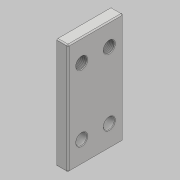
# Autodesk Inventor part: exercise3-3
Saved by Autodesk Inventor 2018 (Build 220112000, 112)
## iProperties
Created: 2020-09-23
Part Number: exercise3-3
Material: 一般
Document SubType Name: Modeling
Designer: 王鼎鈞
Density: 1 g/cm^3
Appearance: 預設
Author: 王鼎鈞
Autodesk Inventor part; units mm, degrees
ref_plane "YZ Plane" through (0, 0, 0) normal (1, 0, 0) x (0, 1, 0)
ref_plane "XZ Plane" through (0, 0, 0) normal (0, 1, 0) x (-1, 0, 0)
ref_plane "XY Plane" through (0, 0, 0) normal (0, 0, 1) x (1, 0, 0)
sketch "草圖1" plane through (0, 0, 0) normal (1, 0, 0) x (0, 1, 0)
  line L0 (-25, 50) -> (25, 50)
  line L1 (25, 50) -> (25, -50)
  line L2 (25, -50) -> (-25, -50)
  line L3 (-25, -50) -> (-25, 50)
  line L4 (-25, 50) -> (25, -50) construction
  line L5 (25, 50) -> (-25, -50) construction
  point P0 (0, 0)
  dimension "d0" = 50
  dimension "d1" = 100
  constraints: 12 end point, 2 midpoint, 2 parallel, 1 horizontal, 1 perpendicular
  measures "d0" distance of L1.end L2.end
  measures "d1" distance of L0.end L1.end
extrude "擠出1" add sketch "草圖1" along normal blind 10
fillet "圓角1" radius 1 4 edges at (5, 25, 50) (5, -25, 50) (5, 25, -50) (5, -25, -50)
chamfer "倒角1" distance 1 angle 45 8 edges at (10, -25, 0) (10, -24.7071, -49.7071) (10, 0, -50) (10, 24.7071, -49.7071) (10, 25, 0) (10, 24.7071, 49.7071) (10, 0, 50) (10, -24.7071, 49.7071)
sketch "草圖2" plane through (10, 0, 0) normal (1, 0, 0) x (0, 0, -1)
  line L0 (-50, 24) -> (-50, -24) projected
  line L1 (49, 25) -> (-49, 25) projected
  line L2 (-30, 24) -> (-30, -24)
  line L3 (50, -24) -> (50, 24) projected
  line L4 (30, -24) -> (30, 24)
  line L5 (30, -12.5) -> (-30, -12.5)
  line L6 (-30, -12.5) -> (-30, 12.5)
  line L7 (-30, 12.5) -> (30, 12.5)
  line L8 (30, 12.5) -> (30, -12.5)
  line L9 (30, -12.5) -> (-30, 12.5) construction
  line L10 (-30, -12.5) -> (30, 12.5) construction
  point P0 (0, 0)
  dimension "d8" = 20
  dimension "d9" = 20
  dimension "d10" = 25
  constraints: 16 end point, 4 coincident, 4 parallel, 2 midpoint, 1 horizontal, 1 perpendicular, 1 point on line
  measures "d8" distance between parallel lines of L0 L2
  measures "d9" distance between parallel lines of L3 L4
  measures "d10" distance of L5.end L6.end
hole "孔1" at (10, 12.5, 30) at (10, -12.5, 30) at (10, 12.5, -30) at (10, -12.5, -30) direction (-1, 0, 0) diameter 10 end through all
thread "螺紋1" size "M10x1.25" class "6H" standard "ANSI Metric M Profile" full length
thread "螺紋2" size "M10x1.5" class "6H" standard "ANSI Metric M Profile" full length
chamfer "倒角2" distance 0.5 angle 45 8 edges at (10, -12.5, -25) (10, 12.5, -25) (10, -12.5, 35) (10, 12.5, 35) (0, -12.5, -25) (0, 12.5, -25) (0, -12.5, 35) (0, 12.5, 35)
